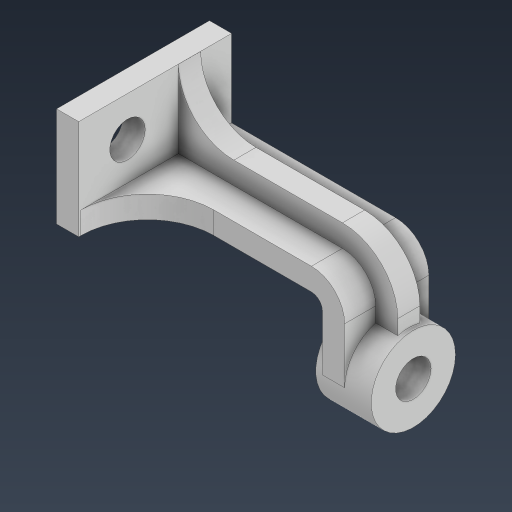
# Autodesk Inventor part: Peça teste 4
Saved by Autodesk Inventor 2024 (Build 280153000, 153)
## iProperties
Created: 2024-02-11
Part Number: Peça teste 4
Material: Genérico
Document SubType Name: Modeling
Designer: Administrator
Density: 1 g/cm^3
Appearance: Padrão
Author: Administrator
Autodesk Inventor part; units mm, degrees
ref_plane "YZ Plane" through (0, 0, 0) normal (1, 0, 0) x (0, 1, 0)
ref_plane "XZ Plane" through (0, 0, 0) normal (0, 1, 0) x (-1, 0, 0)
sketch "Esboço1" plane through (0, 0, 0) normal (1, 0, 0) x (0, 1, 0)
  line L0 (0, 0) -> (45, 0)
  line L1 (45, 0) -> (45, -69)
  line L2 (45, -69) -> (0, -69)
  line L3 (0, -69) -> (0, 0)
  dimension "d0" = 45
  dimension "d1" = 69
  constraints: 8 end point, 2 parallel, 1 horizontal, 1 perpendicular
  measures "d0" distance of L1.end L2.end
  measures "d1" distance of L0.end L1.end
extrude "Extrusão1" add sketch "Esboço1" along normal blind 10
sketch "Esboço2" plane through (10, 0, 0) normal (1, 0, 0) x (0, 0, -1)
  line L0 (69, 45) -> (0, 45) projected
  line L1 (0, 45) -> (0, 0) projected
  point P0 (22, 27)
  dimension "d4" = 18
  dimension "d5" = 22
  measures "d4" distance from line of L0 point (22, 27)
  measures "d5" distance from line of L1 point (22, 27)
hole "Furo1" at (10, 27, -22) direction (-1, 0, 0) diameter 16 end through all
ref_plane "Plano de trabalho1" through (111, 0, 0) normal (1, 0, 0) x (0, 0, -1)
sketch "Esboço3" plane through (111, 0, 0) normal (1, 0, 0) x (0, 0, -1)
  circle A0 centre (50, -30) radius 19
  line L0 (69, 0) -> (69, 45) projected
  line L1 (69, 45) -> (0, 45) projected
  point P0 (0, 0)
  dimension "d14" = 38
  dimension "d15" = 75
  constraints: 1 centre point, 1 tangent
  measures "d14" diameter of A0
  measures "d15" distance from line of L1 A0.centre
extrude "Extrusão2" add sketch "Esboço3" against normal blind 25
sketch "Esboço4" plane through (0, 0, -69) normal (0, 0, -1) x (-1, 0, 0)
  line L0 (-10, 0) -> (-10, 45) construction
  line L1 (-10, 0) -> (-84, 0)
  line L2 (-89, -5) -> (-89, -30)
  line L3 (-89, -30) -> (-99, -30)
  line L4 (-99, -30) -> (-99, -5)
  line L5 (-84, 10) -> (-10, 10)
  line L6 (-111, -11) -> (-111, -49) construction
  line L7 (-111, -30) -> (-86, -30) construction
  line L8 (-86, -49) -> (-86, -11) construction
  arc A0 (-84, 0) -> (-89, -5) centre (-84, -5) ccw
  arc A1 (-84, 10) -> (-99, -5) centre (-84, -5) ccw
  point P0 (0, 0)
  dimension "d18" = 3
  dimension "d19" = 10
  dimension "d20" = 10
  dimension "d21" = 5
  dimension "d22" = 15
  constraints: 12 end point, 4 perpendicular, 4 point on circle, 4 tangent, 2 centre point, 2 midpoint, 2 point on line, 1 horizontal
  measures "d18" distance between parallel lines of L8 L2
  measures "d19" distance between parallel lines of L2 L4
  measures "d20" distance between parallel lines of L1 L5
  measures "d21" radius of A0
  measures "d22" radius of A1
extrude "Extrusão3" add sketch "Esboço4" against normal blind 38 fills toward (-47, 0.05) open curves L1 A0 L2 L3 L4 A1 L5
sketch "Esboço5" plane through (10, 0, 0) normal (1, 0, 0) x (0, 0, -1)
  line L0 (45, 9.9588) -> (55, 9.9588)
  line L1 (55, 9.9588) -> (55, 19.9588)
  line L2 (55, 19.9588) -> (45, 19.9588)
  line L3 (45, 19.9588) -> (45, 9.9588)
  line L4 (31, 10) -> (31, -5) projected
  point P0 (0, 0)
  dimension "d26" = 10
  dimension "d27" = 10
  dimension "d28" = 14
  constraints: 8 end point, 2 parallel, 1 horizontal, 1 perpendicular
  measures "d26" distance of L2.end L1.end
  measures "d27" distance of L1.end L0.end
  measures "d28" distance between parallel lines of L3 L4
sketch3d "Esboço 3D1"
  line L0 (10, 10, -69) -> (84, 10, -69)
  arc A0 (84, 10, -69) -> (99, -5, -69) centre (84, -5, -69) ccw
  line L1 (99, -5, -69) -> (99, -30, -69)
sweep "Varredura1" add profiles "Esboço5" path "Esboço 3D1"
fillet "Arredondamento1" radius 25 1 edges at (10, 19.9588, -50)
fillet "Arredondamento2" radius 30 1 edges at (10, 5, -31)
sketch "Esboço6" plane through (111, -30, -50) normal (1, 0, 0) x (0, 0, -1)
  circle A0 centre (0, 0) radius 19 projected
  point P0 (-50, 30)
  constraints: 1 coincident
hole "Furo2" at (111, -30, -50) direction (-1, 0, 0) diameter 16 end through all
